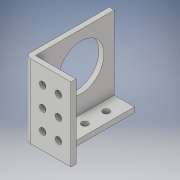
# Autodesk Inventor part: Robot to Bottomish Plate to Pivot Hex Axle OTHER SIDE
Saved by Autodesk Inventor 2017 (Build 210142000, 142)
## iProperties
Created: 2017-06-19
Part Number: Robot to Bottomish Plate to Pivot Hex Axle OTHER SIDE
Material: Generic
Document SubType Name: Modeling
Designer: Matthew
Density: 1 g/cm^3
Appearance: Default
Author: Matthew
Autodesk Inventor part; units mm, degrees
ref_plane "YZ Plane" through (0, 0, 0) normal (1, 0, 0) x (0, 1, 0)
ref_plane "XZ Plane" through (0, 0, 0) normal (0, 1, 0) x (-1, 0, 0)
ref_plane "XY Plane" through (0, 0, 0) normal (0, 0, 1) x (1, 0, 0)
sketch "Sketch1" plane through (0, 0, 0) normal (1, 0, 0) x (0, 1, 0)
  line L0 (0, 0) -> (46.0357, 0)
  line L1 (46.0357, 0) -> (46.0357, -49.1998)
  line L2 (46.0357, -49.1998) -> (0, -49.1998)
  line L3 (0, -49.1998) -> (0, 0)
  circle A0 centre (25.4109, -28.575) radius 14.2748
  point P0 (39.6857, -28.575)
  point P1 (25.4109, -42.8498)
  dimension "d0" = 25.4109
  dimension "d1" = 28.5496
  dimension "d2" = 6.35
  dimension "d3" = 6.35
  dimension "d4" = 28.575
  constraints: 8 end point, 2 parallel, 2 point on circle, 1 centre point, 1 horizontal, 1 horizontal alignment, 1 perpendicular, 1 vertical alignment
  measures "d0" distance from line of L3 A0.centre
  measures "d1" diameter of A0
  measures "d2" distance from line of L1 A0.start
  measures "d3" distance from line of L2 A0.end
  measures "d4" distance from line of L0 A0.centre
extrude "Extrusion1" add sketch "Sketch1" along normal blind 3.175
sketch "Sketch2" plane through (0, 0, -49.1998) normal (0, -1, 0) x (1, 0, 0)
  line L0 (3.175, 49.1998) -> (3.175, 0) projected
  line L1 (3.175, 49.1998) -> (15.875, 49.1998)
  line L2 (15.875, 49.1998) -> (15.875, 0)
  line L3 (15.875, 0) -> (3.175, 0)
  line L4 (3.175, 0) -> (3.175, 49.1998)
  point P0 (0, 49.1998)
  dimension "d7" = 12.7
  constraints: 8 end point, 2 parallel, 1 horizontal, 1 horizontal alignment, 1 perpendicular
  measures "d7" distance of L0.start L1.end
extrude "Extrusion2" add sketch "Sketch2" along normal blind 3.175
sketch "Sketch3" plane through (0, 0, 0) normal (0, 0, 1) x (1, 0, 0)
  line L0 (3.175, 0) -> (3.175, 46.0357) projected
  line L1 (3.175, 0) -> (28.575, 0)
  line L2 (28.575, 0) -> (28.575, 49.2107)
  line L3 (28.575, 49.2107) -> (3.175, 49.2107)
  line L4 (3.175, 49.2107) -> (3.175, 0)
  point P0 (0, 0)
  dimension "d10" = 25.4
  constraints: 8 end point, 2 parallel, 1 horizontal, 1 perpendicular
  measures "d10" distance of L3.end L2.end
extrude "Extrusion3" add sketch "Sketch3" along normal blind 3.175
sketch "Sketch4" plane through (3.175, -3.175, 0) normal (0, 0, 1) x (1, 0, 0)
  line L0 (-3.175, 3.175) -> (0, 3.175) projected
  line L1 (0, 3.175) -> (0, 0) projected
  arc A0 (-3.175, 3.175) -> (0, 0) centre (0, 3.175) ccw
  constraints: 2 point on circle, 1 centre point, 1 coincident
extrude "Extrusion4" add sketch "Sketch4" against normal up to surface (49.1998 mm away)
sketch "Sketch6" plane through (0, 0, 3.175) normal (0, 0, 1) x (1, 0, 0)
  line L0 (3.175, 0) -> (28.575, 0) projected
  line L1 (28.575, 0) -> (28.575, 49.2107) projected
  line L2 (28.575, 49.2107) -> (3.175, 49.2107) projected
  circle A0 centre (10.9643, 35.5428) radius 2.032
  circle A1 centre (20.7857, 35.5428) radius 2.032
  line L3 (12.9963, 35.5428) -> (18.7537, 35.5428)
  line L4 (8.9323, 35.5428) -> (3.175, 35.5428)
  line L5 (22.8177, 35.5428) -> (28.575, 35.5428)
  circle A2 centre (10.9643, 23.0179) radius 2.032
  circle A3 centre (10.9643, 10.4929) radius 2.032
  line L6 (28.575, 49.2107) -> (3.175, 49.2107) projected
  line L7 (10.9643, 25.0499) -> (10.9643, 33.5108)
  line L8 (10.9643, 12.5249) -> (10.9643, 20.9859)
  line L9 (10.9643, 8.4609) -> (10.9643, 0)
  circle A4 centre (20.7857, 23.0179) radius 2.032
  circle A5 centre (20.7857, 10.4929) radius 2.032
  line L10 (3.175, 49.2107) -> (3.175, 0) projected
  line L11 (3.175, 46.0357) -> (28.575, 46.0357)
  line L12 (10.9643, 37.5748) -> (10.9643, 46.0357)
  point P0 (0, 0)
  dimension "d17" = 4.064
  dimension "d20" = 4.064
  dimension "d23" = 4.064
  dimension "d24" = 4.064
  dimension "d25" = 4.064
  dimension "d26" = 4.064
  dimension "d34" = 3.175
  constraints: 16 end point, 10 point on circle, 10 point on line, 8 vertical alignment, 6 centre point, 6 horizontal alignment, 5 collinear, 3 perpendicular, 2 horizontal, 1 vertical
  measures "d17" diameter of A0
  measures "d20" diameter of A1
  measures "d23" diameter of A2
  measures "d24" diameter of A3
  measures "d25" diameter of A4
  measures "d26" diameter of A5
  measures "d34" distance between parallel lines of L2 L11
extrude "Extrusion6" cut sketch "Sketch6" against normal blind 3.175 contours A3 | A0 | A1 | A2 | A4 | A5
sketch "Sketch7" plane through (0, 0, -49.1998) normal (0, 1, 0) x (1, 0, 0)
  line L0 (3.175, -49.1998) -> (15.875, -49.1998) projected
  line L1 (15.875, -49.1998) -> (15.875, 0) construction
  line L2 (15.875, 0) -> (3.175, 0) projected
  line L3 (3.175, -49.1998) -> (3.175, 0) projected
  circle A0 centre (9.525, -11.284) radius 2.032
  circle A1 centre (9.525, -24.5999) radius 2.032
  circle A2 centre (9.525, -37.9158) radius 2.032
  line L4 (9.525, -9.2519) -> (9.525, 0)
  line L5 (9.525, -13.3159) -> (9.525, -22.5679) construction
  line L6 (9.525, -26.6319) -> (9.525, -35.8838)
  line L7 (9.525, -39.9478) -> (9.525, -49.1998)
  line L8 (28.575, -49.1998) -> (3.175, -49.1998) projected
  point P0 (0, -49.1998)
  dimension "d29" = 4.064
  dimension "d30" = 4.064
  dimension "d31" = 4.064
  constraints: 9 vertical alignment, 8 end point, 7 point on line, 6 point on circle, 3 centre point, 3 collinear, 1 midpoint, 1 vertical
  measures "d29" diameter of A0
  measures "d30" diameter of A1
  measures "d31" diameter of A2
extrude "Extrusion7" cut sketch "Sketch7" against normal blind 3.175
sketch "Sketch8" plane through (0, 0, 3.175) normal (0, 0, 1) x (1, 0, 0)
  line L0 (3.175, 49.2107) -> (3.175, 46.0357) projected
  line L1 (28.575, 49.2107) -> (3.175, 49.2107) projected
  line L2 (3.175, 46.0357) -> (28.575, 46.0357)
  line L3 (28.575, 46.0357) -> (28.575, 49.2107)
  line L4 (28.575, 49.2107) -> (3.175, 49.2107)
  line L5 (3.175, 49.2107) -> (3.175, 46.0357)
  point P0 (0, 0)
  constraints: 8 end point, 2 parallel, 1 horizontal, 1 perpendicular
extrude "Extrusion8" cut sketch "Sketch8" against normal blind 25.4
sketch "Sketch9" plane through (0, 46.0357, 0) normal (0, 1, 0) x (1, 0, 0)
  line L0 (0, 0) -> (3.175, 0) projected
  line L1 (3.175, -3.175) -> (3.175, 0) projected
  arc A0 (0, 0) -> (3.175, -3.175) centre (3.175, 0) ccw
  constraints: 2 point on circle, 1 centre point, 1 coincident
extrude "Extrusion9" add sketch "Sketch9" against normal up to surface (46.0357 mm away)
body "Solid1"
